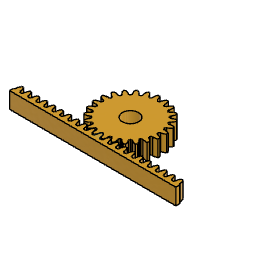
Rack_et_Pinion v6 (Autodesk Fusion 360 design; units mm, degrees)
description: Spur Gear; Module: 2.0; Num Teeth: 24; Pressure Angle: 20.0; Backlash: 0.00 mm
Autodesk Fusion 360 part; units mm, degrees
(part 1 of 3)
sketch "スケッチ1" plane through (0, 0, 0) normal (0, 0, 1) x (1, 0, 0) in component "Spur Gear (24 teeth)"
  circle A0 centre (0, 0) radius 21.5492
  circle A1 centre (0, 0) radius 6.35
extrude "押し出し1" add sketch "スケッチ1" along normal blind 12.7 makes body 1 in component "Spur Gear (24 teeth)"
sketch "スケッチ2" plane through (0, 0, 0) normal (0, 0, 1) x (1, 0, 0) in component "Spur Gear (24 teeth)"
  spline S0 degree 5 poles (22.4799, -1.8102) (22.4899, -1.8111) (22.5101, -1.8124) (22.5404, -1.8137) (22.5808, -1.814) (22.6313, -1.8123) (22.6819, -1.8093) (22.7326, -1.8054) (22.7832, -1.801) (22.8339, -1.7962) (22.8846, -1.7911) (22.9353, -1.7856) (22.986, -1.7795) (23.0367, -1.7727) (23.0874, -1.7652) (23.1381, -1.7571) (23.1889, -1.7484) (23.2396, -1.7393) (23.2903, -1.7297) (23.341, -1.7198) (23.3916, -1.7095) (23.4423, -1.6988) (23.493, -1.6877) (23.5436, -1.6762) (23.5943, -1.6642) (23.6449, -1.6518) (23.6955, -1.6391) (23.7461, -1.6259) (23.7966, -1.6124) (23.8472, -1.5986) (23.8977, -1.5844) (23.9482, -1.5699) (23.9987, -1.555) (24.0491, -1.5398) (24.0996, -1.5242) (24.15, -1.5083) (24.2004, -1.4921) (24.2507, -1.4756) (24.301, -1.4587) (24.3513, -1.4415) (24.4016, -1.424) (24.4518, -1.4062) (24.502, -1.3881) (24.5522, -1.3697) (24.6024, -1.351) (24.6525, -1.3321) (24.7025, -1.3128) (24.7526, -1.2932) (24.8026, -1.2733) (24.8525, -1.2532) (24.9025, -1.2327) (24.9523, -1.212) (25.0022, -1.191) (25.052, -1.1697) (25.1018, -1.1482) (25.1515, -1.1264) (25.2012, -1.1043) (25.2509, -1.0819) (25.3005, -1.0593) (25.35, -1.0364) (25.3995, -1.0133) (25.449, -0.9898) (25.4985, -0.9662) (25.5478, -0.9422) (25.5972, -0.9181) (25.6465, -0.8936) (25.6957, -0.8689) (25.7449, -0.844) (25.7941, -0.8188) (25.8432, -0.7933) (25.8922, -0.7676) (25.9314, -0.7469) (25.9608, -0.7312) (25.9804, -0.7207) (25.9902, -0.7155) knots 0 0 0 0 0 0 0.01428571 0.02857143 0.04285714 0.05714286 0.07142857 0.08571429 0.1 0.11428571 0.12857143 0.14285714 0.15714286 0.17142857 0.18571429 0.2 0.21428571 0.22857143 0.24285714 0.25714286 0.27142857 0.28571429 0.3 0.31428571 0.32857143 0.34285714 0.35714286 0.37142857 0.38571429 0.4 0.41428571 0.42857143 0.44285714 0.45714286 0.47142857 0.48571429 0.5 0.51428571 0.52857143 0.54285714 0.55714286 0.57142857 0.58571429 0.6 0.61428571 0.62857143 0.64285714 0.65714286 0.67142857 0.68571429 0.7 0.71428571 0.72857143 0.74285714 0.75714286 0.77142857 0.78571429 0.8 0.81428571 0.82857143 0.84285714 0.85714286 0.87142857 0.88571429 0.9 0.91428571 0.92857143 0.94285714 0.95714286 0.97142857 0.98571429 1 1 1 1 1 1
  spline S1 degree 5 poles (22.4799, 1.8102) (22.4899, 1.8111) (22.5101, 1.8124) (22.5404, 1.8137) (22.5808, 1.814) (22.6313, 1.8123) (22.6819, 1.8093) (22.7326, 1.8054) (22.7832, 1.801) (22.8339, 1.7962) (22.8846, 1.7911) (22.9353, 1.7856) (22.986, 1.7795) (23.0367, 1.7727) (23.0874, 1.7652) (23.1381, 1.7571) (23.1889, 1.7484) (23.2396, 1.7393) (23.2903, 1.7297) (23.341, 1.7198) (23.3916, 1.7095) (23.4423, 1.6988) (23.493, 1.6877) (23.5436, 1.6762) (23.5943, 1.6642) (23.6449, 1.6518) (23.6955, 1.6391) (23.7461, 1.6259) (23.7966, 1.6124) (23.8472, 1.5986) (23.8977, 1.5844) (23.9482, 1.5699) (23.9987, 1.555) (24.0491, 1.5398) (24.0996, 1.5242) (24.15, 1.5083) (24.2004, 1.4921) (24.2507, 1.4756) (24.301, 1.4587) (24.3513, 1.4415) (24.4016, 1.424) (24.4518, 1.4062) (24.502, 1.3881) (24.5522, 1.3697) (24.6024, 1.351) (24.6525, 1.3321) (24.7025, 1.3128) (24.7526, 1.2932) (24.8026, 1.2733) (24.8525, 1.2532) (24.9025, 1.2327) (24.9523, 1.212) (25.0022, 1.191) (25.052, 1.1697) (25.1018, 1.1482) (25.1515, 1.1264) (25.2012, 1.1043) (25.2509, 1.0819) (25.3005, 1.0593) (25.35, 1.0364) (25.3995, 1.0133) (25.449, 0.9898) (25.4985, 0.9662) (25.5478, 0.9422) (25.5972, 0.9181) (25.6465, 0.8936) (25.6957, 0.8689) (25.7449, 0.844) (25.7941, 0.8188) (25.8432, 0.7933) (25.8922, 0.7676) (25.9314, 0.7469) (25.9608, 0.7312) (25.9804, 0.7207) (25.9902, 0.7155) knots 0 0 0 0 0 0 0.01428571 0.02857143 0.04285714 0.05714286 0.07142857 0.08571429 0.1 0.11428571 0.12857143 0.14285714 0.15714286 0.17142857 0.18571429 0.2 0.21428571 0.22857143 0.24285714 0.25714286 0.27142857 0.28571429 0.3 0.31428571 0.32857143 0.34285714 0.35714286 0.37142857 0.38571429 0.4 0.41428571 0.42857143 0.44285714 0.45714286 0.47142857 0.48571429 0.5 0.51428571 0.52857143 0.54285714 0.55714286 0.57142857 0.58571429 0.6 0.61428571 0.62857143 0.64285714 0.65714286 0.67142857 0.68571429 0.7 0.71428571 0.72857143 0.74285714 0.75714286 0.77142857 0.78571429 0.8 0.81428571 0.82857143 0.84285714 0.85714286 0.87142857 0.88571429 0.9 0.91428571 0.92857143 0.94285714 0.95714286 0.97142857 0.98571429 1 1 1 1 1 1
  arc A0 (25.9902, -0.7155) -> (25.9902, 0.7155) centre (0, 0) ccw
  line L0 (21.4697, -1.7297) -> (22.4799, -1.8102)
  line L1 (21.4697, 1.7297) -> (22.4799, 1.8102)
  line L2 (21.4697, -1.7297) -> (21.4697, 1.7297)
  point P0 (22.7272, -1.8057)
  point P1 (22.9762, -1.7806)
  point P2 (23.2261, -1.7416)
  point P3 (23.4768, -1.6912)
  point P4 (23.7279, -1.6306)
  point P5 (23.9793, -1.5607)
  point P6 (24.231, -1.482)
  point P7 (24.4828, -1.395)
  point P8 (24.7346, -1.3002)
  point P9 (24.9863, -1.1976)
  point P10 (25.2378, -1.0877)
  point P11 (25.489, -0.9706)
  point P12 (25.7398, -0.8465)
  point P13 (22.7272, 1.8057)
  point P14 (22.9762, 1.7806)
  point P15 (23.2261, 1.7416)
  point P16 (23.4768, 1.6912)
  point P17 (23.7279, 1.6306)
  point P18 (23.9793, 1.5607)
  point P19 (24.231, 1.482)
  point P20 (24.4828, 1.395)
  point P21 (24.7346, 1.3002)
  point P22 (24.9863, 1.1976)
  point P23 (25.2378, 1.0877)
  point P24 (25.489, 0.9706)
  point P25 (25.7398, 0.8465)
extrude "押し出し2" add sketch "スケッチ2" along normal blind 12.7 bodies 1 in component "Spur Gear (24 teeth)"
fillet "フィレット1" radius 1 2 edges at (21.4796, -1.7305, 6.35) (21.4796, 1.7305, 6.35) on bodies 1 in component "Spur Gear (24 teeth)"
pattern_circular "C パターン1" count 24 over 360 about axis through (0, 0, 0) along (0, 0, 1) of "押し出し2", "フィレット1" in component "Spur Gear (24 teeth)"
sketch "スケッチ3" plane through (0, 0, 0) normal (0, 0, 1) x (1, 0, 0) in component "Spur Gear (24 teeth)"
  circle A0 centre (0, 0) radius 24 construction
copy_body "ボディのコピーと貼り付け1" bodies 1 makes body 2 in component "Rack"
move_body "移動1" bodies 2 to x (1, 0, 0) y (0, 1, 0) z (0, 0, 1) at (0, -48, 0) in component "Rack"
move_body "移動1'" bodies 1 to x (0.991445, 0.130526, 0) y (-0.130526, 0.991445, 0) z (0, 0, 1) at (0, 0, 0) in component "Spur Gear (24 teeth)"
sketch "スケッチ1 (2)" plane through (0, 0, 12.7) normal (0, 0, 1) x (-1, 0, 0) in component "Rack"
  arc A0 (-21.347, 50.9448) -> (-21.3818, 50.6806) centre (0, 48) ccw
  arc A1 (-22.4535, 49.8082) -> (-21.3818, 50.6806) centre (-22.3741, 50.805) ccw
  line L0 (-22.4535, 49.8082) -> (-22.4799, 49.8102)
  spline S0 degree 5 poles (-22.4799, 49.8102) (-22.4899, 49.8111) (-22.5101, 49.8124) (-22.5404, 49.8137) (-22.5808, 49.814) (-22.6313, 49.8123) (-22.6819, 49.8093) (-22.7326, 49.8054) (-22.7832, 49.801) (-22.8339, 49.7962) (-22.8846, 49.7911) (-22.9353, 49.7856) (-22.986, 49.7795) (-23.0367, 49.7727) (-23.0874, 49.7652) (-23.1381, 49.7571) (-23.1889, 49.7484) (-23.2396, 49.7393) (-23.2903, 49.7297) (-23.341, 49.7198) (-23.3916, 49.7095) (-23.4423, 49.6988) (-23.493, 49.6877) (-23.5436, 49.6762) (-23.5943, 49.6642) (-23.6449, 49.6518) (-23.6955, 49.6391) (-23.7461, 49.6259) (-23.7966, 49.6124) (-23.8472, 49.5986) (-23.8977, 49.5844) (-23.9482, 49.5699) (-23.9987, 49.555) (-24.0491, 49.5398) (-24.0996, 49.5242) (-24.15, 49.5083) (-24.2004, 49.4921) (-24.2507, 49.4756) (-24.301, 49.4587) (-24.3513, 49.4415) (-24.4016, 49.424) (-24.4518, 49.4062) (-24.502, 49.3881) (-24.5522, 49.3697) (-24.6024, 49.351) (-24.6525, 49.3321) (-24.7025, 49.3128) (-24.7526, 49.2932) (-24.8026, 49.2733) (-24.8525, 49.2532) (-24.9025, 49.2327) (-24.9523, 49.212) (-25.0022, 49.191) (-25.052, 49.1697) (-25.1018, 49.1482) (-25.1515, 49.1264) (-25.2012, 49.1043) (-25.2509, 49.0819) (-25.3005, 49.0593) (-25.35, 49.0364) (-25.3995, 49.0133) (-25.449, 48.9898) (-25.4985, 48.9662) (-25.5478, 48.9422) (-25.5972, 48.9181) (-25.6465, 48.8936) (-25.6957, 48.8689) (-25.7449, 48.844) (-25.7941, 48.8188) (-25.8432, 48.7933) (-25.8922, 48.7676) (-25.9314, 48.7469) (-25.9608, 48.7312) (-25.9804, 48.7207) (-25.9902, 48.7155) knots 0 0 0 0 0 0 0.01428571 0.02857143 0.04285714 0.05714286 0.07142857 0.08571429 0.1 0.11428571 0.12857143 0.14285714 0.15714286 0.17142857 0.18571429 0.2 0.21428571 0.22857143 0.24285714 0.25714286 0.27142857 0.28571429 0.3 0.31428571 0.32857143 0.34285714 0.35714286 0.37142857 0.38571429 0.4 0.41428571 0.42857143 0.44285714 0.45714286 0.47142857 0.48571429 0.5 0.51428571 0.52857143 0.54285714 0.55714286 0.57142857 0.58571429 0.6 0.61428571 0.62857143 0.64285714 0.65714286 0.67142857 0.68571429 0.7 0.71428571 0.72857143 0.74285714 0.75714286 0.77142857 0.78571429 0.8 0.81428571 0.82857143 0.84285714 0.85714286 0.87142857 0.88571429 0.9 0.91428571 0.92857143 0.94285714 0.95714286 0.97142857 0.98571429 1 1 1 1 1 1
  arc A2 (-25.9902, 48.7155) -> (-25.9902, 47.2845) centre (0, 48) ccw
  spline S1 degree 5 poles (-25.9902, 47.2845) (-25.9804, 47.2793) (-25.9608, 47.2688) (-25.9314, 47.2531) (-25.8922, 47.2324) (-25.8432, 47.2067) (-25.7941, 47.1812) (-25.7449, 47.156) (-25.6957, 47.1311) (-25.6465, 47.1064) (-25.5972, 47.0819) (-25.5478, 47.0578) (-25.4985, 47.0338) (-25.449, 47.0102) (-25.3995, 46.9867) (-25.35, 46.9636) (-25.3005, 46.9407) (-25.2509, 46.9181) (-25.2012, 46.8957) (-25.1515, 46.8736) (-25.1018, 46.8518) (-25.052, 46.8303) (-25.0022, 46.809) (-24.9523, 46.788) (-24.9025, 46.7673) (-24.8525, 46.7468) (-24.8026, 46.7267) (-24.7526, 46.7068) (-24.7025, 46.6872) (-24.6525, 46.6679) (-24.6024, 46.649) (-24.5522, 46.6303) (-24.502, 46.6119) (-24.4518, 46.5938) (-24.4016, 46.576) (-24.3513, 46.5585) (-24.301, 46.5413) (-24.2507, 46.5244) (-24.2004, 46.5079) (-24.15, 46.4917) (-24.0996, 46.4758) (-24.0491, 46.4602) (-23.9987, 46.445) (-23.9482, 46.4301) (-23.8977, 46.4156) (-23.8472, 46.4014) (-23.7966, 46.3876) (-23.7461, 46.3741) (-23.6955, 46.3609) (-23.6449, 46.3482) (-23.5943, 46.3358) (-23.5436, 46.3238) (-23.493, 46.3123) (-23.4423, 46.3012) (-23.3916, 46.2905) (-23.341, 46.2802) (-23.2903, 46.2703) (-23.2396, 46.2607) (-23.1889, 46.2516) (-23.1381, 46.2429) (-23.0874, 46.2348) (-23.0367, 46.2273) (-22.986, 46.2205) (-22.9353, 46.2144) (-22.8846, 46.2089) (-22.8339, 46.2038) (-22.7832, 46.199) (-22.7326, 46.1946) (-22.6819, 46.1907) (-22.6313, 46.1877) (-22.5808, 46.186) (-22.5404, 46.1863) (-22.5101, 46.1876) (-22.4899, 46.1889) (-22.4799, 46.1898) knots -1 -1 -1 -1 -1 -1 -0.98571429 -0.97142857 -0.95714286 -0.94285714 -0.92857143 -0.91428571 -0.9 -0.88571429 -0.87142857 -0.85714286 -0.84285714 -0.82857143 -0.81428571 -0.8 -0.78571429 -0.77142857 -0.75714286 -0.74285714 -0.72857143 -0.71428571 -0.7 -0.68571429 -0.67142857 -0.65714286 -0.64285714 -0.62857143 -0.61428571 -0.6 -0.58571429 -0.57142857 -0.55714286 -0.54285714 -0.52857143 -0.51428571 -0.5 -0.48571429 -0.47142857 -0.45714286 -0.44285714 -0.42857143 -0.41428571 -0.4 -0.38571429 -0.37142857 -0.35714286 -0.34285714 -0.32857143 -0.31428571 -0.3 -0.28571429 -0.27142857 -0.25714286 -0.24285714 -0.22857143 -0.21428571 -0.2 -0.18571429 -0.17142857 -0.15714286 -0.14285714 -0.12857143 -0.11428571 -0.1 -0.08571429 -0.07142857 -0.05714286 -0.04285714 -0.02857143 -0.01428571 0 0 0 0 0 0
  line L1 (-22.4799, 46.1898) -> (-22.4535, 46.1918)
  arc A3 (-21.3818, 45.3194) -> (-22.4535, 46.1918) centre (-22.3741, 45.195) ccw
  arc A4 (-21.3818, 45.3194) -> (-21.347, 45.0552) centre (0, 48) ccw
  arc A5 (-22.1564, 43.9351) -> (-21.347, 45.0552) centre (-22.3377, 44.9186) ccw
  line L2 (-22.1564, 43.9351) -> (-22.1824, 43.9304)
  spline S2 degree 5 poles (-22.1824, 43.9304) (-22.1923, 43.9285) (-22.2122, 43.9246) (-22.2417, 43.918) (-22.2808, 43.9078) (-22.3292, 43.8932) (-22.3773, 43.8771) (-22.4252, 43.8602) (-22.473, 43.8429) (-22.5207, 43.8252) (-22.5684, 43.8071) (-22.6159, 43.7887) (-22.6633, 43.7696) (-22.7106, 43.75) (-22.7576, 43.7296) (-22.8045, 43.7086) (-22.8512, 43.6871) (-22.8979, 43.6652) (-22.9444, 43.6428) (-22.9908, 43.6201) (-23.037, 43.5971) (-23.0832, 43.5736) (-23.1293, 43.5498) (-23.1752, 43.5255) (-23.221, 43.5008) (-23.2667, 43.4758) (-23.3123, 43.4504) (-23.3578, 43.4246) (-23.4031, 43.3985) (-23.4484, 43.372) (-23.4935, 43.3452) (-23.5385, 43.3181) (-23.5834, 43.2907) (-23.6282, 43.2629) (-23.6729, 43.2349) (-23.7175, 43.2065) (-23.7619, 43.1777) (-23.8063, 43.1487) (-23.8505, 43.1194) (-23.8947, 43.0898) (-23.9387, 43.0599) (-23.9826, 43.0297) (-24.0264, 42.9993) (-24.0701, 42.9685) (-24.1137, 42.9375) (-24.1572, 42.9061) (-24.2006, 42.8745) (-24.2438, 42.8427) (-24.287, 42.8105) (-24.33, 42.7782) (-24.373, 42.7455) (-24.4158, 42.7126) (-24.4585, 42.6794) (-24.5011, 42.6459) (-24.5436, 42.6122) (-24.586, 42.5783) (-24.6283, 42.5441) (-24.6705, 42.5097) (-24.7125, 42.475) (-24.7545, 42.44) (-24.7963, 42.4048) (-24.8381, 42.3694) (-24.8797, 42.3338) (-24.9212, 42.2979) (-24.9626, 42.2617) (-25.0039, 42.2254) (-25.0451, 42.1888) (-25.0861, 42.1519) (-25.1271, 42.1149) (-25.1679, 42.0776) (-25.2086, 42.0401) (-25.2411, 42.0099) (-25.2655, 41.9872) (-25.2816, 41.9719) (-25.2897, 41.9643) knots 0 0 0 0 0 0 0.01428571 0.02857143 0.04285714 0.05714286 0.07142857 0.08571429 0.1 0.11428571 0.12857143 0.14285714 0.15714286 0.17142857 0.18571429 0.2 0.21428571 0.22857143 0.24285714 0.25714286 0.27142857 0.28571429 0.3 0.31428571 0.32857143 0.34285714 0.35714286 0.37142857 0.38571429 0.4 0.41428571 0.42857143 0.44285714 0.45714286 0.47142857 0.48571429 0.5 0.51428571 0.52857143 0.54285714 0.55714286 0.57142857 0.58571429 0.6 0.61428571 0.62857143 0.64285714 0.65714286 0.67142857 0.68571429 0.7 0.71428571 0.72857143 0.74285714 0.75714286 0.77142857 0.78571429 0.8 0.81428571 0.82857143 0.84285714 0.85714286 0.87142857 0.88571429 0.9 0.91428571 0.92857143 0.94285714 0.95714286 0.97142857 0.98571429 1 1 1 1 1 1
  arc A6 (-25.2897, 41.9643) -> (-24.9194, 40.5822) centre (0, 48) ccw
  spline S3 degree 5 poles (-24.9194, 40.5822) (-24.9086, 40.5796) (-24.8869, 40.5745) (-24.8545, 40.567) (-24.8113, 40.5571) (-24.7573, 40.545) (-24.7032, 40.5331) (-24.6492, 40.5215) (-24.5953, 40.5101) (-24.5413, 40.499) (-24.4874, 40.4882) (-24.4335, 40.4776) (-24.3796, 40.4673) (-24.3257, 40.4572) (-24.2718, 40.4474) (-24.218, 40.4378) (-24.1642, 40.4286) (-24.1104, 40.4195) (-24.0567, 40.4108) (-24.003, 40.4023) (-23.9493, 40.3941) (-23.8956, 40.3862) (-23.842, 40.3785) (-23.7884, 40.3711) (-23.7349, 40.364) (-23.6814, 40.3572) (-23.6279, 40.3507) (-23.5744, 40.3444) (-23.521, 40.3385) (-23.4677, 40.3328) (-23.4144, 40.3274) (-23.3611, 40.3223) (-23.3079, 40.3176) (-23.2547, 40.3131) (-23.2016, 40.3089) (-23.1485, 40.305) (-23.0955, 40.3014) (-23.0425, 40.2982) (-22.9896, 40.2952) (-22.9367, 40.2926) (-22.8839, 40.2903) (-22.8312, 40.2883) (-22.7785, 40.2867) (-22.7259, 40.2854) (-22.6733, 40.2844) (-22.6209, 40.2838) (-22.5685, 40.2835) (-22.5161, 40.2835) (-22.4639, 40.2839) (-22.4117, 40.2847) (-22.3596, 40.2859) (-22.3076, 40.2874) (-22.2557, 40.2894) (-22.2039, 40.2917) (-22.1521, 40.2945) (-22.1005, 40.2977) (-22.049, 40.3012) (-21.9975, 40.3052) (-21.9462, 40.3094) (-21.895, 40.3142) (-21.8439, 40.3195) (-21.7929, 40.3254) (-21.7422, 40.3319) (-21.6916, 40.3391) (-21.6412, 40.3469) (-21.591, 40.3551) (-21.5408, 40.3637) (-21.4907, 40.3725) (-21.4408, 40.3818) (-21.3911, 40.392) (-21.3419, 40.4035) (-21.3029, 40.4142) (-21.274, 40.4233) (-21.2549, 40.4298) (-21.2453, 40.4332) knots -1 -1 -1 -1 -1 -1 -0.98571429 -0.97142857 -0.95714286 -0.94285714 -0.92857143 -0.91428571 -0.9 -0.88571429 -0.87142857 -0.85714286 -0.84285714 -0.82857143 -0.81428571 -0.8 -0.78571429 -0.77142857 -0.75714286 -0.74285714 -0.72857143 -0.71428571 -0.7 -0.68571429 -0.67142857 -0.65714286 -0.64285714 -0.62857143 -0.61428571 -0.6 -0.58571429 -0.57142857 -0.55714286 -0.54285714 -0.52857143 -0.51428571 -0.5 -0.48571429 -0.47142857 -0.45714286 -0.44285714 -0.42857143 -0.41428571 -0.4 -0.38571429 -0.37142857 -0.35714286 -0.34285714 -0.32857143 -0.31428571 -0.3 -0.28571429 -0.27142857 -0.25714286 -0.24285714 -0.22857143 -0.21428571 -0.2 -0.18571429 -0.17142857 -0.15714286 -0.14285714 -0.12857143 -0.11428571 -0.1 -0.08571429 -0.07142857 -0.05714286 -0.04285714 -0.02857143 -0.01428571 0 0 0 0 0 0
  line L3 (-21.2453, 40.4332) -> (-21.2205, 40.4421)
  arc A7 (-19.9595, 39.8767) -> (-21.2205, 40.4421) centre (-20.8857, 39.4998) ccw
  arc A8 (-19.9595, 39.8767) -> (-19.8575, 39.6305) centre (0, 48) ccw
  arc A9 (-20.3494, 38.3391) -> (-19.8575, 39.6305) centre (-20.779, 39.2422) ccw
  line L4 (-20.3494, 38.3391) -> (-20.3732, 38.3278)
  spline S4 degree 5 poles (-20.3732, 38.3278) (-20.3824, 38.3235) (-20.4005, 38.3145) (-20.4274, 38.3005) (-20.4625, 38.2806) (-20.5055, 38.2539) (-20.5478, 38.2259) (-20.5897, 38.1972) (-20.6313, 38.1681) (-20.6728, 38.1386) (-20.7142, 38.1089) (-20.7554, 38.0787) (-20.7962, 38.0481) (-20.8367, 38.0168) (-20.8769, 37.985) (-20.9168, 37.9526) (-20.9563, 37.9197) (-20.9957, 37.8865) (-21.0348, 37.8529) (-21.0738, 37.8189) (-21.1125, 37.7847) (-21.1511, 37.7501) (-21.1894, 37.7151) (-21.2275, 37.6798) (-21.2653, 37.6441) (-21.303, 37.6081) (-21.3404, 37.5717) (-21.3777, 37.5351) (-21.4147, 37.4981) (-21.4516, 37.4608) (-21.4882, 37.4233) (-21.5247, 37.3854) (-21.561, 37.3473) (-21.5971, 37.3089) (-21.633, 37.2702) (-21.6687, 37.2313) (-21.7042, 37.192) (-21.7395, 37.1525) (-21.7747, 37.1127) (-21.8096, 37.0727) (-21.8444, 37.0325) (-21.879, 36.9919) (-21.9135, 36.9512) (-21.9477, 36.9101) (-21.9818, 36.8689) (-22.0157, 36.8274) (-22.0494, 36.7856) (-22.0829, 36.7436) (-22.1163, 36.7014) (-22.1495, 36.659) (-22.1825, 36.6163) (-22.2154, 36.5735) (-22.248, 36.5303) (-22.2805, 36.487) (-22.3129, 36.4435) (-22.345, 36.3997) (-22.377, 36.3557) (-22.4088, 36.3115) (-22.4405, 36.2671) (-22.472, 36.2225) (-22.5033, 36.1777) (-22.5344, 36.1327) (-22.5654, 36.0875) (-22.5962, 36.0421) (-22.6268, 35.9965) (-22.6573, 35.9507) (-22.6876, 35.9046) (-22.7177, 35.8584) (-22.7477, 35.812) (-22.7775, 35.7655) (-22.8071, 35.7187) (-22.8307, 35.6811) (-22.8483, 35.6529) (-22.86, 35.634) (-22.8659, 35.6245) knots 0 0 0 0 0 0 0.01428571 0.02857143 0.04285714 0.05714286 0.07142857 0.08571429 0.1 0.11428571 0.12857143 0.14285714 0.15714286 0.17142857 0.18571429 0.2 0.21428571 0.22857143 0.24285714 0.25714286 0.27142857 0.28571429 0.3 0.31428571 0.32857143 0.34285714 0.35714286 0.37142857 0.38571429 0.4 0.41428571 0.42857143 0.44285714 0.45714286 0.47142857 0.48571429 0.5 0.51428571 0.52857143 0.54285714 0.55714286 0.57142857 0.58571429 0.6 0.61428571 0.62857143 0.64285714 0.65714286 0.67142857 0.68571429 0.7 0.71428571 0.72857143 0.74285714 0.75714286 0.77142857 0.78571429 0.8 0.81428571 0.82857143 0.84285714 0.85714286 0.87142857 0.88571429 0.9 0.91428571 0.92857143 0.94285714 0.95714286 0.97142857 0.98571429 1 1 1 1 1 1
  arc A10 (-22.8659, 35.6245) -> (-22.1504, 34.3853) centre (0, 48) ccw
  spline S5 degree 5 poles (-22.1504, 34.3853) (-22.1393, 34.3857) (-22.1171, 34.3863) (-22.0838, 34.3875) (-22.0395, 34.3891) (-21.9842, 34.3914) (-21.9289, 34.3939) (-21.8738, 34.3966) (-21.8187, 34.3996) (-21.7637, 34.4029) (-21.7088, 34.4064) (-21.654, 34.4101) (-21.5992, 34.414) (-21.5446, 34.4183) (-21.49, 34.4227) (-21.4356, 34.4274) (-21.3812, 34.4324) (-21.3269, 34.4376) (-21.2727, 34.4431) (-21.2187, 34.4488) (-21.1647, 34.4547) (-21.1108, 34.461) (-21.057, 34.4675) (-21.0034, 34.4742) (-20.9498, 34.4812) (-20.8963, 34.4885) (-20.843, 34.496) (-20.7898, 34.5038) (-20.7366, 34.5118) (-20.6836, 34.5202) (-20.6307, 34.5288) (-20.578, 34.5377) (-20.5253, 34.5468) (-20.4728, 34.5562) (-20.4204, 34.5659) (-20.3681, 34.5759) (-20.316, 34.5862) (-20.264, 34.5968) (-20.2121, 34.6076) (-20.1603, 34.6188) (-20.1087, 34.6302) (-20.0573, 34.6419) (-20.006, 34.654) (-19.9548, 34.6663) (-19.9038, 34.679) (-19.853, 34.692) (-19.8023, 34.7053) (-19.7517, 34.7189) (-19.7014, 34.7328) (-19.6512, 34.747) (-19.6011, 34.7616) (-19.5513, 34.7766) (-19.5017, 34.7919) (-19.4522, 34.8076) (-19.403, 34.8237) (-19.354, 34.8401) (-19.3051, 34.8569) (-19.2564, 34.874) (-19.2079, 34.8914) (-19.1597, 34.9092) (-19.1117, 34.9276) (-19.064, 34.9464) (-19.0167, 34.9659) (-18.9697, 34.986) (-18.9231, 35.0065) (-18.8766, 35.0275) (-18.8304, 35.0487) (-18.7843, 35.0702) (-18.7385, 35.0921) (-18.6931, 35.1148) (-18.6485, 35.1387) (-18.6137, 35.1591) (-18.5881, 35.1754) (-18.5713, 35.1866) (-18.563, 35.1924) knots -1 -1 -1 -1 -1 -1 -0.98571429 -0.97142857 -0.95714286 -0.94285714 -0.92857143 -0.91428571 -0.9 -0.88571429 -0.87142857 -0.85714286 -0.84285714 -0.82857143 -0.81428571 -0.8 -0.78571429 -0.77142857 -0.75714286 -0.74285714 -0.72857143 -0.71428571 -0.7 -0.68571429 -0.67142857 -0.65714286 -0.64285714 -0.62857143 -0.61428571 -0.6 -0.58571429 -0.57142857 -0.55714286 -0.54285714 -0.52857143 -0.51428571 -0.5 -0.48571429 -0.47142857 -0.45714286 -0.44285714 -0.42857143 -0.41428571 -0.4 -0.38571429 -0.37142857 -0.35714286 -0.34285714 -0.32857143 -0.31428571 -0.3 -0.28571429 -0.27142857 -0.25714286 -0.24285714 -0.22857143 -0.21428571 -0.2 -0.18571429 -0.17142857 -0.15714286 -0.14285714 -0.12857143 -0.11428571 -0.1 -0.08571429 -0.07142857 -0.05714286 -0.04285714 -0.02857143 -0.01428571 0 0 0 0 0 0
  line L5 (-18.563, 35.1924) -> (-18.5413, 35.2073)
  arc A11 (-17.1769, 34.9876) -> (-18.5413, 35.2073) centre (-17.974, 34.3838) ccw
  arc A12 (-17.1769, 34.9876) -> (-17.0147, 34.7762) centre (0, 48) ccw
  arc A13 (-17.1556, 33.4015) -> (-17.0147, 34.7762) centre (-17.8043, 34.1626) ccw
  line L6 (-17.1556, 33.4015) -> (-17.1757, 33.3844)
  spline S6 degree 5 poles (-17.1757, 33.3844) (-17.1834, 33.3778) (-17.1986, 33.3645) (-17.2209, 33.344) (-17.2497, 33.3157) (-17.2843, 33.2788) (-17.3179, 33.2408) (-17.3509, 33.2023) (-17.3836, 33.1633) (-17.4161, 33.1241) (-17.4484, 33.0847) (-17.4803, 33.0449) (-17.5119, 33.0047) (-17.5429, 32.9641) (-17.5735, 32.9229) (-17.6036, 32.8813) (-17.6333, 32.8393) (-17.6627, 32.797) (-17.6918, 32.7544) (-17.7206, 32.7115) (-17.7492, 32.6684) (-17.7775, 32.625) (-17.8054, 32.5813) (-17.8331, 32.5374) (-17.8604, 32.4931) (-17.8875, 32.4486) (-17.9142, 32.4037) (-17.9407, 32.3587) (-17.9669, 32.3134) (-17.9929, 32.2679) (-18.0186, 32.2221) (-18.044, 32.1761) (-18.0692, 32.1299) (-18.0941, 32.0835) (-18.1188, 32.0368) (-18.1432, 31.9899) (-18.1673, 31.9428) (-18.1912, 31.8955) (-18.2149, 31.848) (-18.2383, 31.8003) (-18.2615, 31.7524) (-18.2844, 31.7043) (-18.3071, 31.656) (-18.3296, 31.6075) (-18.3518, 31.5588) (-18.3738, 31.51) (-18.3956, 31.4609) (-18.4171, 31.4117) (-18.4384, 31.3623) (-18.4595, 31.3127) (-18.4804, 31.263) (-18.501, 31.213) (-18.5214, 31.1629) (-18.5416, 31.1127) (-18.5615, 31.0623) (-18.5813, 31.0117) (-18.6008, 30.9609) (-18.6201, 30.91) (-18.6392, 30.8589) (-18.658, 30.8077) (-18.6767, 30.7563) (-18.6951, 30.7047) (-18.7133, 30.6531) (-18.7313, 30.6012) (-18.7491, 30.5492) (-18.7667, 30.4971) (-18.784, 30.4448) (-18.8012, 30.3924) (-18.8181, 30.3398) (-18.8348, 30.2871) (-18.8514, 30.2342) (-18.8644, 30.1919) (-18.8741, 30.16) (-18.8805, 30.1387) (-18.8837, 30.1281) knots 0 0 0 0 0 0 0.01428571 0.02857143 0.04285714 0.05714286 0.07142857 0.08571429 0.1 0.11428571 0.12857143 0.14285714 0.15714286 0.17142857 0.18571429 0.2 0.21428571 0.22857143 0.24285714 0.25714286 0.27142857 0.28571429 0.3 0.31428571 0.32857143 0.34285714 0.35714286 0.37142857 0.38571429 0.4 0.41428571 0.42857143 0.44285714 0.45714286 0.47142857 0.48571429 0.5 0.51428571 0.52857143 0.54285714 0.55714286 0.57142857 0.58571429 0.6 0.61428571 0.62857143 0.64285714 0.65714286 0.67142857 0.68571429 0.7 0.71428571 0.72857143 0.74285714 0.75714286 0.77142857 0.78571429 0.8 0.81428571 0.82857143 0.84285714 0.85714286 0.87142857 0.88571429 0.9 0.91428571 0.92857143 0.94285714 0.95714286 0.97142857 0.98571429 1 1 1 1 1 1
  arc A14 (-18.8837, 30.1281) -> (-17.8719, 29.1163) centre (0, 48) ccw
  spline S7 degree 5 poles (-17.8719, 29.1163) (-17.8613, 29.1195) (-17.84, 29.1259) (-17.8081, 29.1356) (-17.7658, 29.1486) (-17.7129, 29.1652) (-17.6602, 29.1819) (-17.6076, 29.1988) (-17.5552, 29.216) (-17.5029, 29.2333) (-17.4508, 29.2509) (-17.3988, 29.2687) (-17.3469, 29.2867) (-17.2953, 29.3049) (-17.2437, 29.3233) (-17.1923, 29.342) (-17.1411, 29.3608) (-17.09, 29.3799) (-17.0391, 29.3992) (-16.9883, 29.4187) (-16.9377, 29.4385) (-16.8873, 29.4584) (-16.8371, 29.4786) (-16.787, 29.499) (-16.737, 29.5196) (-16.6873, 29.5405) (-16.6377, 29.5616) (-16.5883, 29.5829) (-16.5391, 29.6044) (-16.49, 29.6262) (-16.4412, 29.6482) (-16.3925, 29.6704) (-16.344, 29.6929) (-16.2957, 29.7156) (-16.2476, 29.7385) (-16.1997, 29.7617) (-16.152, 29.7851) (-16.1045, 29.8088) (-16.0572, 29.8327) (-16.0101, 29.8568) (-15.9632, 29.8812) (-15.9165, 29.9059) (-15.8701, 29.9308) (-15.8239, 29.956) (-15.7779, 29.9814) (-15.7321, 30.0071) (-15.6866, 30.0331) (-15.6413, 30.0593) (-15.5963, 30.0858) (-15.5514, 30.1125) (-15.5069, 30.1396) (-15.4626, 30.1669) (-15.4187, 30.1946) (-15.375, 30.2225) (-15.3316, 30.2508) (-15.2885, 30.2794) (-15.2456, 30.3082) (-15.203, 30.3373) (-15.1607, 30.3667) (-15.1187, 30.3964) (-15.0771, 30.4265) (-15.0359, 30.4571) (-14.9953, 30.4881) (-14.9551, 30.5197) (-14.9153, 30.5516) (-14.8759, 30.5839) (-14.8367, 30.6164) (-14.7977, 30.6491) (-14.7592, 30.6821) (-14.7212, 30.7157) (-14.6843, 30.7503) (-14.656, 30.7791) (-14.6355, 30.8014) (-14.6222, 30.8166) (-14.6156, 30.8243) knots -1 -1 -1 -1 -1 -1 -0.98571429 -0.97142857 -0.95714286 -0.94285714 -0.92857143 -0.91428571 -0.9 -0.88571429 -0.87142857 -0.85714286 -0.84285714 -0.82857143 -0.81428571 -0.8 -0.78571429 -0.77142857 -0.75714286 -0.74285714 -0.72857143 -0.71428571 -0.7 -0.68571429 -0.67142857 -0.65714286 -0.64285714 -0.62857143 -0.61428571 -0.6 -0.58571429 -0.57142857 -0.55714286 -0.54285714 -0.52857143 -0.51428571 -0.5 -0.48571429 -0.47142857 -0.45714286 -0.44285714 -0.42857143 -0.41428571 -0.4 -0.38571429 -0.37142857 -0.35714286 -0.34285714 -0.32857143 -0.31428571 -0.3 -0.28571429 -0.27142857 -0.25714286 -0.24285714 -0.22857143 -0.21428571 -0.2 -0.18571429 -0.17142857 -0.15714286 -0.14285714 -0.12857143 -0.11428571 -0.1 -0.08571429 -0.07142857 -0.05714286 -0.04285714 -0.02857143 -0.01428571 0 0 0 0 0 0
  line L7 (-14.6156, 30.8243) -> (-14.5985, 30.8444)
  arc A15 (-13.2238, 30.9853) -> (-14.5985, 30.8444) centre (-13.8374, 30.1957) ccw
  arc A16 (-13.2238, 30.9853) -> (-13.0124, 30.8231) centre (0, 48) ccw
  arc A17 (-12.7927, 29.4587) -> (-13.0124, 30.8231) centre (-13.6162, 30.026) ccw
  line L8 (-12.7927, 29.4587) -> (-12.8076, 29.437)
  spline S8 degree 5 poles (-12.8076, 29.437) (-12.8134, 29.4287) (-12.8246, 29.4119) (-12.8409, 29.3863) (-12.8613, 29.3515) (-12.8852, 29.3069) (-12.9079, 29.2615) (-12.9298, 29.2157) (-12.9513, 29.1696) (-12.9725, 29.1234) (-12.9935, 29.0769) (-13.014, 29.0303) (-13.0341, 28.9833) (-13.0536, 28.936) (-13.0724, 28.8883) (-13.0908, 28.8403) (-13.1086, 28.7921) (-13.126, 28.7436) (-13.1431, 28.6949) (-13.1599, 28.646) (-13.1763, 28.597) (-13.1924, 28.5478) (-13.2081, 28.4983) (-13.2234, 28.4487) (-13.2384, 28.3989) (-13.253, 28.3488) (-13.2672, 28.2986) (-13.2811, 28.2483) (-13.2947, 28.1977) (-13.308, 28.147) (-13.321, 28.0962) (-13.3337, 28.0452) (-13.346, 27.994) (-13.3581, 27.9427) (-13.3698, 27.8913) (-13.3812, 27.8397) (-13.3924, 27.7879) (-13.4032, 27.736) (-13.4138, 27.684) (-13.4241, 27.6319) (-13.4341, 27.5796) (-13.4438, 27.5272) (-13.4532, 27.4747) (-13.4623, 27.422) (-13.4712, 27.3693) (-13.4798, 27.3164) (-13.4882, 27.2634) (-13.4962, 27.2102) (-13.504, 27.157) (-13.5115, 27.1037) (-13.5188, 27.0502) (-13.5258, 26.9966) (-13.5325, 26.943) (-13.539, 26.8892) (-13.5453, 26.8353) (-13.5512, 26.7813) (-13.5569, 26.7273) (-13.5624, 26.6731) (-13.5676, 26.6188) (-13.5726, 26.5644) (-13.5773, 26.51) (-13.5817, 26.4554) (-13.586, 26.4008) (-13.5899, 26.346) (-13.5936, 26.2912) (-13.5971, 26.2363) (-13.6004, 26.1813) (-13.6034, 26.1262) (-13.6061, 26.0711) (-13.6086, 26.0158) (-13.6109, 25.9605) (-13.6125, 25.9162) (-13.6137, 25.8829) (-13.6143, 25.8607) (-13.6147, 25.8496) knots 0 0 0 0 0 0 0.01428571 0.02857143 0.04285714 0.05714286 0.07142857 0.08571429 0.1 0.11428571 0.12857143 0.14285714 0.15714286 0.17142857 0.18571429 0.2 0.21428571 0.22857143 0.24285714 0.25714286 0.27142857 0.28571429 0.3 0.31428571 0.32857143 0.34285714 0.35714286 0.37142857 0.38571429 0.4 0.41428571 0.42857143 0.44285714 0.45714286 0.47142857 0.48571429 0.5 0.51428571 0.52857143 0.54285714 0.55714286 0.57142857 0.58571429 0.6 0.61428571 0.62857143 0.64285714 0.65714286 0.67142857 0.68571429 0.7 0.71428571 0.72857143 0.74285714 0.75714286 0.77142857 0.78571429 0.8 0.81428571 0.82857143 0.84285714 0.85714286 0.87142857 0.88571429 0.9 0.91428571 0.92857143 0.94285714 0.95714286 0.97142857 0.98571429 1 1 1 1 1 1
  arc A18 (-13.6147, 25.8496) -> (-12.3755, 25.1341) centre (0, 48) ccw
  spline S9 degree 5 poles (-12.3755, 25.1341) (-12.366, 25.14) (-12.3471, 25.1517) (-12.3189, 25.1693) (-12.2813, 25.1929) (-12.2345, 25.2225) (-12.188, 25.2523) (-12.1416, 25.2823) (-12.0954, 25.3124) (-12.0493, 25.3427) (-12.0035, 25.3732) (-11.9579, 25.4038) (-11.9125, 25.4346) (-11.8673, 25.4656) (-11.8223, 25.4967) (-11.7775, 25.528) (-11.7329, 25.5595) (-11.6885, 25.5912) (-11.6443, 25.623) (-11.6003, 25.655) (-11.5565, 25.6871) (-11.513, 25.7195) (-11.4697, 25.752) (-11.4265, 25.7846) (-11.3837, 25.8175) (-11.341, 25.8505) (-11.2986, 25.8837) (-11.2564, 25.9171) (-11.2144, 25.9506) (-11.1726, 25.9843) (-11.1311, 26.0182) (-11.0899, 26.0523) (-11.0488, 26.0865) (-11.0081, 26.121) (-10.9675, 26.1556) (-10.9273, 26.1904) (-10.8873, 26.2253) (-10.8475, 26.2605) (-10.808, 26.2958) (-10.7687, 26.3313) (-10.7298, 26.367) (-10.6911, 26.4029) (-10.6527, 26.439) (-10.6146, 26.4753) (-10.5767, 26.5118) (-10.5392, 26.5484) (-10.5019, 26.5853) (-10.4649, 26.6223) (-10.4283, 26.6596) (-10.3919, 26.697) (-10.3559, 26.7347) (-10.3202, 26.7725) (-10.2849, 26.8106) (-10.2499, 26.8489) (-10.2153, 26.8875) (-10.1811, 26.9262) (-10.1471, 26.9652) (-10.1135, 27.0043) (-10.0803, 27.0437) (-10.0474, 27.0832) (-10.015, 27.1231) (-9.9832, 27.1633) (-9.9519, 27.2038) (-9.9213, 27.2446) (-9.8911, 27.2858) (-9.8614, 27.3272) (-9.8319, 27.3687) (-9.8028, 27.4103) (-9.7741, 27.4522) (-9.7461, 27.4945) (-9.7194, 27.5375) (-9.6995, 27.5726) (-9.6855, 27.5995) (-9.6765, 27.6176) (-9.6722, 27.6268) knots -1 -1 -1 -1 -1 -1 -0.98571429 -0.97142857 -0.95714286 -0.94285714 -0.92857143 -0.91428571 -0.9 -0.88571429 -0.87142857 -0.85714286 -0.84285714 -0.82857143 -0.81428571 -0.8 -0.78571429 -0.77142857 -0.75714286 -0.74285714 -0.72857143 -0.71428571 -0.7 -0.68571429 -0.67142857 -0.65714286 -0.64285714 -0.62857143 -0.61428571 -0.6 -0.58571429 -0.57142857 -0.55714286 -0.54285714 -0.52857143 -0.51428571 -0.5 -0.48571429 -0.47142857 -0.45714286 -0.44285714 -0.42857143 -0.41428571 -0.4 -0.38571429 -0.37142857 -0.35714286 -0.34285714 -0.32857143 -0.31428571 -0.3 -0.28571429 -0.27142857 -0.25714286 -0.24285714 -0.22857143 -0.21428571 -0.2 -0.18571429 -0.17142857 -0.15714286 -0.14285714 -0.12857143 -0.11428571 -0.1 -0.08571429 -0.07142857 -0.05714286 -0.04285714 -0.02857143 -0.01428571 0 0 0 0 0 0
  line L9 (-9.6722, 27.6268) -> (-9.6609, 27.6506)
  arc A19 (-8.3695, 28.1425) -> (-9.6609, 27.6506) centre (-8.7578, 27.221) ccw
  arc A20 (-8.3695, 28.1425) -> (-8.1233, 28.0405) centre (0, 48) ccw
  arc A21 (-7.5579, 26.7795) -> (-8.1233, 28.0405) centre (-8.5002, 27.1143) ccw
  line L10 (-7.5579, 26.7795) -> (-7.5668, 26.7547)
  spline S10 degree 5 poles (-7.5668, 26.7547) (-7.5702, 26.7451) (-7.5767, 26.726) (-7.5858, 26.6971) (-7.5965, 26.6581) (-7.608, 26.6089) (-7.6182, 26.5592) (-7.6275, 26.5093) (-7.6363, 26.4592) (-7.6449, 26.409) (-7.6531, 26.3588) (-7.6609, 26.3084) (-7.6681, 26.2578) (-7.6746, 26.2071) (-7.6805, 26.1561) (-7.6858, 26.105) (-7.6906, 26.0538) (-7.6948, 26.0025) (-7.6988, 25.951) (-7.7023, 25.8995) (-7.7055, 25.8479) (-7.7083, 25.7961) (-7.7106, 25.7443) (-7.7126, 25.6924) (-7.7141, 25.6404) (-7.7153, 25.5883) (-7.7161, 25.5361) (-7.7165, 25.4839) (-7.7165, 25.4315) (-7.7162, 25.3791) (-7.7156, 25.3267) (-7.7146, 25.2741) (-7.7133, 25.2215) (-7.7117, 25.1688) (-7.7097, 25.1161) (-7.7074, 25.0633) (-7.7048, 25.0104) (-7.7018, 24.9575) (-7.6986, 24.9045) (-7.695, 24.8515) (-7.6911, 24.7984) (-7.6869, 24.7453) (-7.6824, 24.6921) (-7.6777, 24.6389) (-7.6726, 24.5856) (-7.6672, 24.5323) (-7.6615, 24.479) (-7.6556, 24.4256) (-7.6493, 24.3721) (-7.6428, 24.3186) (-7.636, 24.2651) (-7.6289, 24.2116) (-7.6215, 24.158) (-7.6138, 24.1044) (-7.6059, 24.0507) (-7.5977, 23.997) (-7.5892, 23.9433) (-7.5805, 23.8896) (-7.5714, 23.8358) (-7.5622, 23.782) (-7.5526, 23.7282) (-7.5428, 23.6743) (-7.5327, 23.6204) (-7.5224, 23.5665) (-7.5118, 23.5126) (-7.501, 23.4587) (-7.4899, 23.4047) (-7.4785, 23.3508) (-7.4669, 23.2968) (-7.455, 23.2427) (-7.4429, 23.1887) (-7.433, 23.1455) (-7.4255, 23.1131) (-7.4204, 23.0914) (-7.4178, 23.0806) knots 0 0 0 0 0 0 0.01428571 0.02857143 0.04285714 0.05714286 0.07142857 0.08571429 0.1 0.11428571 0.12857143 0.14285714 0.15714286 0.17142857 0.18571429 0.2 0.21428571 0.22857143 0.24285714 0.25714286 0.27142857 0.28571429 0.3 0.31428571 0.32857143 0.34285714 0.35714286 0.37142857 0.38571429 0.4 0.41428571 0.42857143 0.44285714 0.45714286 0.47142857 0.48571429 0.5 0.51428571 0.52857143 0.54285714 0.55714286 0.57142857 0.58571429 0.6 0.61428571 0.62857143 0.64285714 0.65714286 0.67142857 0.68571429 0.7 0.71428571 0.72857143 0.74285714 0.75714286 0.77142857 0.78571429 0.8 0.81428571 0.82857143 0.84285714 0.85714286 0.87142857 0.88571429 0.9 0.91428571 0.92857143 0.94285714 0.95714286 0.97142857 0.98571429 1 1 1 1 1 1
  arc A22 (-7.4178, 23.0806) -> (-6.0357, 22.7103) centre (0, 48) ccw
  spline S11 degree 5 poles (-6.0357, 22.7103) (-6.0281, 22.7184) (-6.0128, 22.7345) (-5.9901, 22.7589) (-5.9599, 22.7914) (-5.9224, 22.8321) (-5.8851, 22.8729) (-5.8481, 22.9139) (-5.8112, 22.9549) (-5.7746, 22.9961) (-5.7383, 23.0374) (-5.7021, 23.0788) (-5.6662, 23.1203) (-5.6306, 23.1619) (-5.5952, 23.2037) (-5.56, 23.2455) (-5.525, 23.2875) (-5.4903, 23.3295) (-5.4559, 23.3717) (-5.4217, 23.414) (-5.3878, 23.4564) (-5.3541, 23.4989) (-5.3206, 23.5415) (-5.2874, 23.5842) (-5.2545, 23.627) (-5.2218, 23.67) (-5.1895, 23.713) (-5.1573, 23.7562) (-5.1255, 23.7994) (-5.0939, 23.8428) (-5.0625, 23.8863) (-5.0315, 23.9299) (-5.0007, 23.9736) (-4.9703, 24.0174) (-4.9401, 24.0613) (-4.9102, 24.1053) (-4.8806, 24.1495) (-4.8513, 24.1937) (-4.8223, 24.2381) (-4.7935, 24.2825) (-4.7651, 24.3271) (-4.7371, 24.3718) (-4.7093, 24.4166) (-4.6819, 24.4615) (-4.6548, 24.5065) (-4.628, 24.5516) (-4.6015, 24.5969) (-4.5754, 24.6422) (-4.5496, 24.6877) (-4.5242, 24.7333) (-4.4992, 24.779) (-4.4745, 24.8248) (-4.4502, 24.8707) (-4.4264, 24.9168) (-4.4029, 24.963) (-4.3799, 25.0092) (-4.3572, 25.0556) (-4.3348, 25.1021) (-4.3129, 25.1488) (-4.2914, 25.1955) (-4.2704, 25.2424) (-4.25, 25.2894) (-4.2304, 25.3367) (-4.2113, 25.3841) (-4.1929, 25.4316) (-4.1748, 25.4793) (-4.1571, 25.527) (-4.1398, 25.5748) (-4.1229, 25.6227) (-4.1068, 25.6708) (-4.0922, 25.7192) (-4.082, 25.7583) (-4.0754, 25.7878) (-4.0715, 25.8077) (-4.0696, 25.8176) knots -1 -1 -1 -1 -1 -1 -0.98571429 -0.97142857 -0.95714286 -0.94285714 -0.92857143 -0.91428571 -0.9 -0.88571429 -0.87142857 -0.85714286 -0.84285714 -0.82857143 -0.81428571 -0.8 -0.78571429 -0.77142857 -0.75714286 -0.74285714 -0.72857143 -0.71428571 -0.7 -0.68571429 -0.67142857 -0.65714286 -0.64285714 -0.62857143 -0.61428571 -0.6 -0.58571429 -0.57142857 -0.55714286 -0.54285714 -0.52857143 -0.51428571 -0.5 -0.48571429 -0.47142857 -0.45714286 -0.44285714 -0.42857143 -0.41428571 -0.4 -0.38571429 -0.37142857 -0.35714286 -0.34285714 -0.32857143 -0.31428571 -0.3 -0.28571429 -0.27142857 -0.25714286 -0.24285714 -0.22857143 -0.21428571 -0.2 -0.18571429 -0.17142857 -0.15714286 -0.14285714 -0.12857143 -0.11428571 -0.1 -0.08571429 -0.07142857 -0.05714286 -0.04285714 -0.02857143 -0.01428571 0 0 0 0 0 0
  line L11 (-4.0696, 25.8176) -> (-4.0649, 25.8436)
  arc A23 (-2.9448, 26.653) -> (-4.0649, 25.8436) centre (-3.0814, 25.6623) ccw
  arc A24 (-2.9448, 26.653) -> (-2.6806, 26.6182) centre (0, 48) ccw
  arc A25 (-1.8082, 25.5465) -> (-2.6806, 26.6182) centre (-2.805, 25.6259) ccw
  line L12 (-1.8082, 25.5465) -> (-1.8102, 25.5201)
  spline S12 degree 5 poles (-1.8102, 25.5201) (-1.8111, 25.5101) (-1.8124, 25.4899) (-1.8137, 25.4596) (-1.814, 25.4192) (-1.8123, 25.3687) (-1.8093, 25.3181) (-1.8054, 25.2674) (-1.801, 25.2168) (-1.7962, 25.1661) (-1.7911, 25.1154) (-1.7856, 25.0647) (-1.7795, 25.014) (-1.7727, 24.9633) (-1.7652, 24.9126) (-1.7571, 24.8619) (-1.7484, 24.8111) (-1.7393, 24.7604) (-1.7297, 24.7097) (-1.7198, 24.659) (-1.7095, 24.6084) (-1.6988, 24.5577) (-1.6877, 24.507) (-1.6762, 24.4564) (-1.6642, 24.4057) (-1.6518, 24.3551) (-1.6391, 24.3045) (-1.6259, 24.2539) (-1.6124, 24.2034) (-1.5986, 24.1528) (-1.5844, 24.1023) (-1.5699, 24.0518) (-1.555, 24.0013) (-1.5398, 23.9509) (-1.5242, 23.9004) (-1.5083, 23.85) (-1.4921, 23.7996) (-1.4756, 23.7493) (-1.4587, 23.699) (-1.4415, 23.6487) (-1.424, 23.5984) (-1.4062, 23.5482) (-1.3881, 23.498) (-1.3697, 23.4478) (-1.351, 23.3976) (-1.3321, 23.3475) (-1.3128, 23.2975) (-1.2932, 23.2474) (-1.2733, 23.1974) (-1.2532, 23.1475) (-1.2327, 23.0975) (-1.212, 23.0477) (-1.191, 22.9978) (-1.1697, 22.948) (-1.1482, 22.8982) (-1.1264, 22.8485) (-1.1043, 22.7988) (-1.0819, 22.7491) (-1.0593, 22.6995) (-1.0364, 22.65) (-1.0133, 22.6005) (-0.9898, 22.551) (-0.9662, 22.5015) (-0.9422, 22.4522) (-0.9181, 22.4028) (-0.8936, 22.3535) (-0.8689, 22.3043) (-0.844, 22.2551) (-0.8188, 22.2059) (-0.7933, 22.1568) (-0.7676, 22.1078) (-0.7469, 22.0686) (-0.7312, 22.0392) (-0.7207, 22.0196) (-0.7155, 22.0098) knots 0 0 0 0 0 0 0.01428571 0.02857143 0.04285714 0.05714286 0.07142857 0.08571429 0.1 0.11428571 0.12857143 0.14285714 0.15714286 0.17142857 0.18571429 0.2 0.21428571 0.22857143 0.24285714 0.25714286 0.27142857 0.28571429 0.3 0.31428571 0.32857143 0.34285714 0.35714286 0.37142857 0.38571429 0.4 0.41428571 0.42857143 0.44285714 0.45714286 0.47142857 0.48571429 0.5 0.51428571 0.52857143 0.54285714 0.55714286 0.57142857 0.58571429 0.6 0.61428571 0.62857143 0.64285714 0.65714286 0.67142857 0.68571429 0.7 0.71428571 0.72857143 0.74285714 0.75714286 0.77142857 0.78571429 0.8 0.81428571 0.82857143 0.84285714 0.85714286 0.87142857 0.88571429 0.9 0.91428571 0.92857143 0.94285714 0.95714286 0.97142857 0.98571429 1 1 1 1 1 1
  arc A26 (-0.7155, 22.0098) -> (0.7155, 22.0098) centre (0, 48) ccw
  spline S13 degree 5 poles (0.7155, 22.0098) (0.7207, 22.0196) (0.7312, 22.0392) (0.7469, 22.0686) (0.7676, 22.1078) (0.7933, 22.1568) (0.8188, 22.2059) (0.844, 22.2551) (0.8689, 22.3043) (0.8936, 22.3535) (0.9181, 22.4028) (0.9422, 22.4522) (0.9662, 22.5015) (0.9898, 22.551) (1.0133, 22.6005) (1.0364, 22.65) (1.0593, 22.6995) (1.0819, 22.7491) (1.1043, 22.7988) (1.1264, 22.8485) (1.1482, 22.8982) (1.1697, 22.948) (1.191, 22.9978) (1.212, 23.0477) (1.2327, 23.0975) (1.2532, 23.1475) (1.2733, 23.1974) (1.2932, 23.2474) (1.3128, 23.2975) (1.3321, 23.3475) (1.351, 23.3976) (1.3697, 23.4478) (1.3881, 23.498) (1.4062, 23.5482) (1.424, 23.5984) (1.4415, 23.6487) (1.4587, 23.699) (1.4756, 23.7493) (1.4921, 23.7996) (1.5083, 23.85) (1.5242, 23.9004) (1.5398, 23.9509) (1.555, 24.0013) (1.5699, 24.0518) (1.5844, 24.1023) (1.5986, 24.1528) (1.6124, 24.2034) (1.6259, 24.2539) (1.6391, 24.3045) (1.6518, 24.3551) (1.6642, 24.4057) (1.6762, 24.4564) (1.6877, 24.507) (1.6988, 24.5577) (1.7095, 24.6084) (1.7198, 24.659) (1.7297, 24.7097) (1.7393, 24.7604) (1.7484, 24.8111) (1.7571, 24.8619) (1.7652, 24.9126) (1.7727, 24.9633) (1.7795, 25.014) (1.7856, 25.0647) (1.7911, 25.1154) (1.7962, 25.1661) (1.801, 25.2168) (1.8054, 25.2674) (1.8093, 25.3181) (1.8123, 25.3687) (1.814, 25.4192) (1.8137, 25.4596) (1.8124, 25.4899) (1.8111, 25.5101) (1.8102, 25.5201) knots -1 -1 -1 -1 -1 -1 -0.98571429 -0.97142857 -0.95714286 -0.94285714 -0.92857143 -0.91428571 -0.9 -0.88571429 -0.87142857 -0.85714286 -0.84285714 -0.82857143 -0.81428571 -0.8 -0.78571429 -0.77142857 -0.75714286 -0.74285714 -0.72857143 -0.71428571 -0.7 -0.68571429 -0.67142857 -0.65714286 -0.64285714 -0.62857143 -0.61428571 -0.6 -0.58571429 -0.57142857 -0.55714286 -0.54285714 -0.52857143 -0.51428571 -0.5 -0.48571429 -0.47142857 -0.45714286 -0.44285714 -0.42857143 -0.41428571 -0.4 -0.38571429 -0.37142857 -0.35714286 -0.34285714 -0.32857143 -0.31428571 -0.3 -0.28571429 -0.27142857 -0.25714286 -0.24285714 -0.22857143 -0.21428571 -0.2 -0.18571429 -0.17142857 -0.15714286 -0.14285714 -0.12857143 -0.11428571 -0.1 -0.08571429 -0.07142857 -0.05714286 -0.04285714 -0.02857143 -0.01428571 0 0 0 0 0 0
  line L13 (1.8102, 25.5201) -> (1.8082, 25.5465)
  arc A27 (2.6806, 26.6182) -> (1.8082, 25.5465) centre (2.805, 25.6259) ccw
  arc A28 (2.6806, 26.6182) -> (2.9448, 26.653) centre (0, 48) ccw
  arc A29 (4.0649, 25.8436) -> (2.9448, 26.653) centre (3.0814, 25.6623) ccw
  line L14 (4.0649, 25.8436) -> (4.0696, 25.8176)
  spline S14 degree 5 poles (4.0696, 25.8176) (4.0715, 25.8077) (4.0754, 25.7878) (4.082, 25.7583) (4.0922, 25.7192) (4.1068, 25.6708) (4.1229, 25.6227) (4.1398, 25.5748) (4.1571, 25.527) (4.1748, 25.4793) (4.1929, 25.4316) (4.2113, 25.3841) (4.2304, 25.3367) (4.25, 25.2894) (4.2704, 25.2424) (4.2914, 25.1955) (4.3129, 25.1488) (4.3348, 25.1021) (4.3572, 25.0556) (4.3799, 25.0092) (4.4029, 24.963) (4.4264, 24.9168) (4.4502, 24.8707) (4.4745, 24.8248) (4.4992, 24.779) (4.5242, 24.7333) (4.5496, 24.6877) (4.5754, 24.6422) (4.6015, 24.5969) (4.628, 24.5516) (4.6548, 24.5065) (4.6819, 24.4615) (4.7093, 24.4166) (4.7371, 24.3718) (4.7651, 24.3271) (4.7935, 24.2825) (4.8223, 24.2381) (4.8513, 24.1937) (4.8806, 24.1495) (4.9102, 24.1053) (4.9401, 24.0613) (4.9703, 24.0174) (5.0007, 23.9736) (5.0315, 23.9299) (5.0625, 23.8863) (5.0939, 23.8428) (5.1255, 23.7994) (5.1573, 23.7562) (5.1895, 23.713) (5.2218, 23.67) (5.2545, 23.627) (5.2874, 23.5842) (5.3206, 23.5415) (5.3541, 23.4989) (5.3878, 23.4564) (5.4217, 23.414) (5.4559, 23.3717) (5.4903, 23.3295) (5.525, 23.2875) (5.56, 23.2455) (5.5952, 23.2037) (5.6306, 23.1619) (5.6662, 23.1203) (5.7021, 23.0788) (5.7383, 23.0374) (5.7746, 22.9961) (5.8112, 22.9549) (5.8481, 22.9139) (5.8851, 22.8729) (5.9224, 22.8321) (5.9599, 22.7914) (5.9901, 22.7589) (6.0128, 22.7345) (6.0281, 22.7184) (6.0357, 22.7103) knots 0 0 0 0 0 0 0.01428571 0.02857143 0.04285714 0.05714286 0.07142857 0.08571429 0.1 0.11428571 0.12857143 0.14285714 0.15714286 0.17142857 0.18571429 0.2 0.21428571 0.22857143 0.24285714 0.25714286 0.27142857 0.28571429 0.3 0.31428571 0.32857143 0.34285714 0.35714286 0.37142857 0.38571429 0.4 0.41428571 0.42857143 0.44285714 0.45714286 0.47142857 0.48571429 0.5 0.51428571 0.52857143 0.54285714 0.55714286 0.57142857 0.58571429 0.6 0.61428571 0.62857143 0.64285714 0.65714286 0.67142857 0.68571429 0.7 0.71428571 0.72857143 0.74285714 0.75714286 0.77142857 0.78571429 0.8 0.81428571 0.82857143 0.84285714 0.85714286 0.87142857 0.88571429 0.9 0.91428571 0.92857143 0.94285714 0.95714286 0.97142857 0.98571429 1 1 1 1 1 1
  arc A30 (6.0357, 22.7103) -> (7.4178, 23.0806) centre (0, 48) ccw
  spline S15 degree 5 poles (7.4178, 23.0806) (7.4204, 23.0914) (7.4255, 23.1131) (7.433, 23.1455) (7.4429, 23.1887) (7.455, 23.2427) (7.4669, 23.2968) (7.4785, 23.3508) (7.4899, 23.4047) (7.501, 23.4587) (7.5118, 23.5126) (7.5224, 23.5665) (7.5327, 23.6204) (7.5428, 23.6743) (7.5526, 23.7282) (7.5622, 23.782) (7.5714, 23.8358) (7.5805, 23.8896) (7.5892, 23.9433) (7.5977, 23.997) (7.6059, 24.0507) (7.6138, 24.1044) (7.6215, 24.158) (7.6289, 24.2116) (7.636, 24.2651) (7.6428, 24.3186) (7.6493, 24.3721) (7.6556, 24.4256) (7.6615, 24.479) (7.6672, 24.5323) (7.6726, 24.5856) (7.6777, 24.6389) (7.6824, 24.6921) (7.6869, 24.7453) (7.6911, 24.7984) (7.695, 24.8515) (7.6986, 24.9045) (7.7018, 24.9575) (7.7048, 25.0104) (7.7074, 25.0633) (7.7097, 25.1161) (7.7117, 25.1688) (7.7133, 25.2215) (7.7146, 25.2741) (7.7156, 25.3267) (7.7162, 25.3791) (7.7165, 25.4315) (7.7165, 25.4839) (7.7161, 25.5361) (7.7153, 25.5883) (7.7141, 25.6404) (7.7126, 25.6924) (7.7106, 25.7443) (7.7083, 25.7961) (7.7055, 25.8479) (7.7023, 25.8995) (7.6988, 25.951) (7.6948, 26.0025) (7.6906, 26.0538) (7.6858, 26.105) (7.6805, 26.1561) (7.6746, 26.2071) (7.6681, 26.2578) (7.6609, 26.3084) (7.6531, 26.3588) (7.6449, 26.409) (7.6363, 26.4592) (7.6275, 26.5093) (7.6182, 26.5592) (7.608, 26.6089) (7.5965, 26.6581) (7.5858, 26.6971) (7.5767, 26.726) (7.5702, 26.7451) (7.5668, 26.7547) knots -1 -1 -1 -1 -1 -1 -0.98571429 -0.97142857 -0.95714286 -0.94285714 -0.92857143 -0.91428571 -0.9 -0.88571429 -0.87142857 -0.85714286 -0.84285714 -0.82857143 -0.81428571 -0.8 -0.78571429 -0.77142857 -0.75714286 -0.74285714 -0.72857143 -0.71428571 -0.7 -0.68571429 -0.67142857 -0.65714286 -0.64285714 -0.62857143 -0.61428571 -0.6 -0.58571429 -0.57142857 -0.55714286 -0.54285714 -0.52857143 -0.51428571 -0.5 -0.48571429 -0.47142857 -0.45714286 -0.44285714 -0.42857143 -0.41428571 -0.4 -0.38571429 -0.37142857 -0.35714286 -0.34285714 -0.32857143 -0.31428571 -0.3 -0.28571429 -0.27142857 -0.25714286 -0.24285714 -0.22857143 -0.21428571 -0.2 -0.18571429 -0.17142857 -0.15714286 -0.14285714 -0.12857143 -0.11428571 -0.1 -0.08571429 -0.07142857 -0.05714286 -0.04285714 -0.02857143 -0.01428571 0 0 0 0 0 0
  line L15 (7.5668, 26.7547) -> (7.5579, 26.7795)
  arc A31 (8.1233, 28.0405) -> (7.5579, 26.7795) centre (8.5002, 27.1143) ccw
  arc A32 (8.1233, 28.0405) -> (8.3695, 28.1425) centre (0, 48) ccw
  arc A33 (9.6609, 27.6506) -> (8.3695, 28.1425) centre (8.7578, 27.221) ccw
  line L16 (9.6609, 27.6506) -> (9.6722, 27.6268)
  spline S16 degree 5 poles (9.6722, 27.6268) (9.6765, 27.6176) (9.6855, 27.5995) (9.6995, 27.5726) (9.7194, 27.5375) (9.7461, 27.4945) (9.7741, 27.4522) (9.8028, 27.4103) (9.8319, 27.3687) (9.8614, 27.3272) (9.8911, 27.2858) (9.9213, 27.2446) (9.9519, 27.2038) (9.9832, 27.1633) (10.015, 27.1231) (10.0474, 27.0832) (10.0803, 27.0437) (10.1135, 27.0043) (10.1471, 26.9652) (10.1811, 26.9262) (10.2153, 26.8875) (10.2499, 26.8489) (10.2849, 26.8106) (10.3202, 26.7725) (10.3559, 26.7347) (10.3919, 26.697) (10.4283, 26.6596) (10.4649, 26.6223) (10.5019, 26.5853) (10.5392, 26.5484) (10.5767, 26.5118) (10.6146, 26.4753) (10.6527, 26.439) (10.6911, 26.4029) (10.7298, 26.367) (10.7687, 26.3313) (10.808, 26.2958) (10.8475, 26.2605) (10.8873, 26.2253) (10.9273, 26.1904) (10.9675, 26.1556) (11.0081, 26.121) (11.0488, 26.0865) (11.0899, 26.0523) (11.1311, 26.0182) (11.1726, 25.9843) (11.2144, 25.9506) (11.2564, 25.9171) (11.2986, 25.8837) (11.341, 25.8505) (11.3837, 25.8175) (11.4265, 25.7846) (11.4697, 25.752) (11.513, 25.7195) (11.5565, 25.6871) (11.6003, 25.655) (11.6443, 25.623) (11.6885, 25.5912) (11.7329, 25.5595) (11.7775, 25.528) (11.8223, 25.4967) (11.8673, 25.4656) (11.9125, 25.4346) (11.9579, 25.4038) (12.0035, 25.3732) (12.0493, 25.3427) (12.0954, 25.3124) (12.1416, 25.2823) (12.188, 25.2523) (12.2345, 25.2225) (12.2813, 25.1929) (12.3189, 25.1693) (12.3471, 25.1517) (12.366, 25.14) (12.3755, 25.1341) knots 0 0 0 0 0 0 0.01428571 0.02857143 0.04285714 0.05714286 0.07142857 0.08571429 0.1 0.11428571 0.12857143 0.14285714 0.15714286 0.17142857 0.18571429 0.2 0.21428571 0.22857143 0.24285714 0.25714286 0.27142857 0.28571429 0.3 0.31428571 0.32857143 0.34285714 0.35714286 0.37142857 0.38571429 0.4 0.41428571 0.42857143 0.44285714 0.45714286 0.47142857 0.48571429 0.5 0.51428571 0.52857143 0.54285714 0.55714286 0.57142857 0.58571429 0.6 0.61428571 0.62857143 0.64285714 0.65714286 0.67142857 0.68571429 0.7 0.71428571 0.72857143 0.74285714 0.75714286 0.77142857 0.78571429 0.8 0.81428571 0.82857143 0.84285714 0.85714286 0.87142857 0.88571429 0.9 0.91428571 0.92857143 0.94285714 0.95714286 0.97142857 0.98571429 1 1 1 1 1 1
  arc A34 (12.3755, 25.1341) -> (13.6147, 25.8496) centre (0, 48) ccw